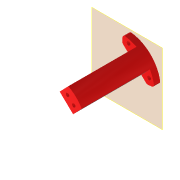
# Autodesk Inventor part: IM_Matchboxscope_Laserholder
Saved by Autodesk Inventor 2022 (Build 260153000, 153)
## iProperties
Created: 2023-05-17
Part Number: IM_Matchboxscope_Laserholder
Material: Generisch
Document SubType Name: Modeling
Designer: diederichbenedict
Density: 1 g/cm^3
Appearance: Glatt - Rot
Author: diederichbenedict
Autodesk Inventor part; units mm, degrees
ref_plane "YZ Plane" through (0, 0, 0) normal (1, 0, 0) x (0, 1, 0)
ref_plane "XZ Plane" through (0, 0, 0) normal (0, 1, 0) x (-1, 0, 0)
ref_plane "XY Plane" through (0, 0, 0) normal (0, 0, 1) x (1, 0, 0)
ref_plane "Arbeitsebene1" through (0, 0, 0) normal (0, 0, 1) x (1, 0, 0)
sketch "Skizze1" plane through (0, 0, 0) normal (0, 0, 1) x (1, 0, 0)
  circle A0 centre (-8.37, 7.9978) radius 1.4 projected
  circle A1 centre (8.3745, -8.0022) radius 1.4 projected
  spline S0 degree 2 poles (24.1427, 2.2394) (24.731, 1.8489) (25.3785, 0.5587) (25.3785, -0.3311) knots 0 0 0 1 2 2 2 projected
  spline S1 degree 2 poles (25.3785, -0.3311) (25.3785, -1.1665) (24.7013, -2.5111) (24.1328, -2.8868) knots 0 0 0 1 2 2 2 projected
  spline S2 degree 2 poles (24.1328, -2.8868) (23.6682, -3.1784) (22.7141, -3.3761) (21.9726, -3.3761) knots 0 0 0 1 2 2 2 projected
  line L0 (21.9726, -3.3761) -> (20.5687, -3.3761) projected
  line L1 (20.5687, -3.3761) -> (20.5687, 2.7239) projected
  line L2 (20.5687, 2.7239) -> (21.9578, 2.7239) projected
  spline S3 degree 2 poles (21.9578, 2.7239) (22.8179, 2.7239) (23.7967, 2.4668) (24.1427, 2.2394) knots 0 0 0 1 2 2 2 projected
  spline S4 degree 2 poles (19.1896, -2.9312) (18.8979, -3.1982) (18.1564, -3.4849) (17.5978, -3.4849) knots 0 0 0 1 2 2 2 projected
  spline S5 degree 2 poles (17.5978, -3.4849) (16.9354, -3.4849) (16.0061, -3.2081) (15.5958, -3.0103) knots 0 0 0 1 2 2 2 projected
  line L3 (15.5958, -3.0103) -> (15.5958, -1.992) projected
  line L4 (15.5958, -1.992) -> (15.6551, -1.992) projected
  spline S6 degree 2 poles (15.6551, -1.992) (16.0555, -2.3677) (17.0689, -2.783) (17.5385, -2.783) knots 0 0 0 1 2 2 2 projected
  spline S7 degree 2 poles (17.5385, -2.783) (18.2108, -2.783) (18.8979, -2.2244) (18.8979, -1.7646) knots 0 0 0 1 2 2 2 projected
  spline S8 degree 2 poles (18.8979, -1.7646) (18.8979, -1.3988) (18.5371, -0.9441) (18.1465, -0.8304) knots 0 0 0 1 2 2 2 projected
  spline S9 degree 2 poles (18.1465, -0.8304) (17.8648, -0.7513) (17.3952, -0.6425) (17.0442, -0.5535) knots 0 0 0 1 2 2 2 projected
  spline S10 degree 2 poles (17.0442, -0.5535) (16.7278, -0.4695) (16.2285, -0.2174) (16.0358, -0.0147) knots 0 0 0 1 2 2 2 projected
  spline S11 degree 2 poles (16.0358, -0.0147) (15.8479, 0.188) (15.6403, 0.7317) (15.6403, 1.0876) knots 0 0 0 1 2 2 2 projected
  spline S12 degree 2 poles (15.6403, 1.0876) (15.6403, 1.8291) (16.797, 2.8326) (17.6918, 2.8326) knots 0 0 0 1 2 2 2 projected
  spline S13 degree 2 poles (17.6918, 2.8326) (18.2059, 2.8326) (19.1154, 2.6299) (19.5059, 2.4371) knots 0 0 0 1 2 2 2 projected
  line L5 (19.5059, 2.4371) -> (19.5059, 1.4683) projected
  line L6 (19.5059, 1.4683) -> (19.4466, 1.4683) projected
  spline S14 degree 2 poles (19.4466, 1.4683) (19.155, 1.7352) (18.2454, 2.1307) (17.7461, 2.1307) knots 0 0 0 1 2 2 2 projected
  spline S15 degree 2 poles (17.7461, 2.1307) (17.1826, 2.1307) (16.4856, 1.6017) (16.4856, 1.1717) knots 0 0 0 1 2 2 2 projected
  spline S16 degree 2 poles (16.4856, 1.1717) (16.4856, 0.7861) (16.8959, 0.3264) (17.2815, 0.2226) knots 0 0 0 1 2 2 2 projected
  spline S17 degree 2 poles (17.2815, 0.2226) (17.5385, 0.1534) (18.285, -0.0246) (18.5321, -0.0988) knots 0 0 0 1 2 2 2 projected
  spline S18 degree 2 poles (18.5321, -0.0988) (19.1599, -0.2915) (19.7432, -1.0676) (19.7432, -1.6361) knots 0 0 0 1 2 2 2 projected
  spline S19 degree 2 poles (19.7432, -1.6361) (19.7432, -1.997) (19.4516, -2.689) (19.1896, -2.9312) knots 0 0 0 1 2 2 2 projected
  line L7 (-17.7002, -6.4434) -> (-23.8502, -6.4434) projected
  arc A2 (-23.8502, -6.4434) -> (-24.8892, -7.3274) centre (-23.8502, -7.496) ccw projected
  arc A3 (-25.1732, 6.2825) -> (-24.8892, -7.3274) centre (0, 0) ccw projected
  arc A4 (-25.1732, 6.2825) -> (-24.1417, 5.4391) centre (-24.1417, 6.4917) ccw projected
  line L8 (-24.1417, 5.4391) -> (-17.7002, 5.4391) projected
  arc A5 (-15.7528, 3.4917) -> (-17.7002, 5.4391) centre (-17.7002, 3.4917) ccw projected
  line L9 (-15.7528, 3.4917) -> (-15.7528, -4.496) projected
  arc A6 (-17.7002, -6.4434) -> (-15.7528, -4.496) centre (-17.7002, -4.496) ccw projected
  circle A7 centre (0, 0) radius 25.963 projected
  circle A8 centre (-16.3217, -17.1216) radius 2.05 projected
  circle A9 centre (6.1284, 23.0203) radius 2.05 projected
  circle A10 centre (22.752, 7.1358) radius 2.05 projected
  circle A11 centre (-9.4998, -11.0022) radius 4 projected
  circle A12 centre (0.0001, -0.0022) radius 7.5 projected
  circle A13 centre (0, 0) radius 26.963
  circle A14 centre (0, 0) radius 20.963
  line L10 (1.3131, 26.931) -> (1.0209, 20.9381)
  line L11 (20.8731, 1.9397) -> (26.8473, 2.4948)
  circle A15 centre (6.1284, 23.0203) radius 1.5
  circle A16 centre (22.752, 7.1358) radius 1.5
  line L12 (1.0209, 20.9381) -> (20.8731, 1.9397)
  point P0 (0, 0)
  point P1 (20.7853, 2.7239)
  point P2 (24.1373, 2.243)
  point P3 (20.5687, 2.2309)
  dimension "d0" = 1
  dimension "d1" = 6
  dimension "d2" = 5
  dimension "d3" = 5
  dimension "d6" = 3
  dimension "d7" = 3
  constraints: 6 end point, 4 centre point, 4 point on circle, 2 coincident, 2 line through centre
  measures "d0" radial gap between concentric circles of A7 A13
  measures "d1" radial gap between concentric circles of A13 A14
  measures "d2" distance from line of L10 A9.centre
  measures "d3" distance from line of L11 A10.centre
  measures "d6" diameter of A15
  measures "d7" diameter of A16
extrude "Extrusion1" add sketch "Skizze1" along normal blind 5 contours L11 A14 L2 S3 | S3 L2 A14 L10 A7 L11 | L12 L1 L2 A14 | A7 L10 A13 L11 | L2 L1 L12 A14 | A9 | A10 picked at (11.3891, 23.8845)
fillet "Rundung1" radius 2 4 edges at (1.0209, 20.9381, 2.5) (1.3131, 26.931, 2.5) (20.8731, 1.9397, 2.5) (26.8473, 2.4948, 2.5)
sketch "Skizze2" plane through (0, 0, 5) normal (0, 0, 1) x (1, 0, 0)
  arc A0 (24.776, 2.3024) -> (26.5611, 4.6378) centre (24.5909, 4.2938) ccw projected
  arc A1 (26.5611, 4.6378) -> (3.4665, 26.7392) centre (0, 0) ccw projected
  arc A2 (3.4665, 26.7392) -> (1.2118, 24.8532) centre (3.2094, 24.7558) ccw projected
  line L0 (1.2118, 24.8532) -> (1.0653, 21.8495) projected
  arc A3 (1.0653, 21.8495) -> (1.6802, 20.3072) centre (3.063, 21.7521) ccw projected
  line L1 (1.6802, 20.3072) -> (20.2138, 2.5706) projected
  arc A4 (20.2138, 2.5706) -> (21.7817, 2.0241) centre (21.5966, 4.0155) ccw projected
  line L2 (21.7817, 2.0241) -> (24.776, 2.3024) projected
  circle A5 centre (6.1284, 23.0203) radius 1.5 projected
  circle A6 centre (22.752, 7.1358) radius 1.5 projected
  line L3 (1.6802, 20.3072) -> (20.2138, 2.5706) projected
  line L4 (5.5366, 16.6166) -> (12.4984, 23.8913)
  line L5 (16.3684, 6.2506) -> (23.3271, 13.5221)
  point P0 (0, 0)
  dimension "d9" = 4
  dimension "d10" = 4
  constraints: 4 end point, 3 perpendicular, 2 point on circle, 2 point on line
  measures "d9" distance from line of L4 A5.centre
  measures "d10" distance from line of A6.centre L5
extrude "Extrusion2" add sketch "Skizze2" along normal blind 55 contours L5 L1 L4 A1
sketch "Skizze3" plane through (0, 0, 60) normal (0, 0, 1) x (1, 0, 0)
  arc A0 (23.3271, 13.5221) -> (12.4984, 23.8913) centre (0, 0) ccw projected
  line L0 (12.4984, 23.8913) -> (5.5366, 16.6166) projected
  line L1 (5.5366, 16.6166) -> (16.3684, 6.2506) projected
  line L2 (16.3684, 6.2506) -> (23.3271, 13.5221) projected
  circle A1 centre (11.8835, 17.4634) radius 1.4
  circle A2 centre (16.9355, 12.6286) radius 1.4
  point P0 (0, 0)
  dimension "d13" = 2.8
  dimension "d14" = 2.8
  dimension "d15" = 4
  dimension "d16" = 4
  dimension "d17" = 5
  dimension "d18" = 5
  constraints: 2 centre point
  measures "d13" diameter of A1
  measures "d14" diameter of A2
  measures "d15" distance from line of A1.centre L0
  measures "d16" distance from line of L2 A2.centre
  measures "d17" distance from line of L1 A2.centre
  measures "d18" distance from line of L1 A1.centre
extrude "Extrusion3" cut sketch "Skizze3" against normal blind 20 contours A1 | A2
